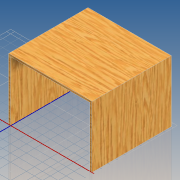
# Autodesk Inventor part: Tunnel
Saved by Autodesk Inventor 2020 (Build 240168000, 168)
## iProperties
Created: 2019-11-19
Part Number: Tunnel
Material: Generic
Document SubType Name: Modeling
Designer: Berkant
Density: 1 g/cm^3
Appearance: Default
Author: Berkant
Autodesk Inventor part; units mm, degrees
ref_plane "YZ Plane" through (0, 0, 0) normal (1, 0, 0) x (0, 1, 0)
ref_plane "XZ Plane" through (0, 0, 0) normal (0, 1, 0) x (-1, 0, 0)
ref_plane "XY Plane" through (0, 0, 0) normal (0, 0, 1) x (1, 0, 0)
sketch "Sketch1" plane through (0, 0, 0) normal (0, 0, 1) x (1, 0, 0)
  line L0 (0, 0) -> (400, 0)
  line L1 (400, 0) -> (400, 300)
  line L2 (400, 300) -> (0, 300)
  line L3 (0, 300) -> (0, 0)
  line L4 (0, 0) -> (-10, 0)
  line L5 (-10, 0) -> (410, 0)
  line L6 (410, 0) -> (410, 310)
  line L7 (410, 310) -> (-10, 310)
  line L8 (-10, 310) -> (-10, 0)
  dimension "d0" = 400
  dimension "d1" = 300
  dimension "d4" = 10
  constraints: 18 end point, 4 parallel, 3 horizontal, 2 perpendicular
  measures "d0" distance of L2.end L1.end
  measures "d1" distance of L1.end L0.end
  measures "d4" distance of L0.start L4.end
extrude "Extrusion1" add sketch "Sketch1" against normal blind 400
extrude "Extrusion2" cut sketch "Sketch1" against normal blind 400 contours L3 L2 L1 L0
body "Solid1"
